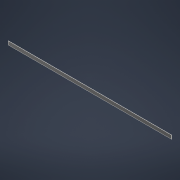
# Autodesk Inventor part: LuggageStrapShort
Saved by Autodesk Inventor 2021 (Build 250183000, 183)
## iProperties
Created: 2021-01-31
Part Number: LuggageStrapShort
Material: Generic
Document SubType Name: Modeling
Designer: argon
Density: 1 g/cm^3
Appearance: Fine Textured - Black
Author: argon
Autodesk Inventor part; units mm, degrees
ref_plane "YZ Plane" through (0, 0, 0) normal (1, 0, 0) x (0, 1, 0)
ref_plane "XZ Plane" through (0, 0, 0) normal (0, 1, 0) x (-1, 0, 0)
ref_plane "XY Plane" through (0, 0, 0) normal (0, 0, 1) x (1, 0, 0)
sketch "Sketch1" plane through (0, 0, 0) normal (0, 0, 1) x (1, 0, 0)
  line L0 (-1635, 36) -> (1635, 36)
  line L1 (1635, 36) -> (1635, -36)
  line L2 (1635, -36) -> (-1635, -36)
  line L3 (-1635, -36) -> (-1635, 36)
  line L4 (-1635, 36) -> (1635, -36) construction
  line L5 (1635, 36) -> (-1635, -36) construction
  point P0 (0, 0)
  dimension "d0" = 3270
  dimension "d1" = 72
  constraints: 12 end point, 2 midpoint, 2 parallel, 1 horizontal, 1 perpendicular
  measures "d0" distance of L0.start L0.end
  measures "d1" distance of L0.end L1.end
extrude "Extrusion1" add sketch "Sketch1" along normal blind 5
body "Solid1"
